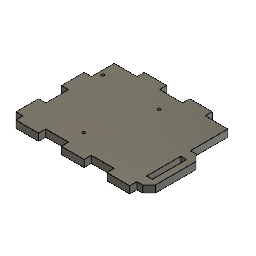
Right Side (Autodesk Fusion 360 design; units mm, degrees)
Autodesk Fusion 360 part; units mm, degrees
sketch "Sketch1" plane through (0, 0, 0) normal (0, 1, 0) x (1, 0, 0)
  line L0 (100, 38.5) -> (105, 38.5)
  line L1 (105, 38.5) -> (105, 8.5)
  line L2 (105, 8.5) -> (100, 8.5)
  line L3 (100, 8.5) -> (100, 38.5)
  line L4 (100, 0) -> (105, 0)
  line L5 (105, 0) -> (110.6569, 5.6569)
  line L6 (100, 47) -> (105, 47)
  line L7 (105, 47) -> (110.6569, 41.3431)
  line L8 (110.6569, 41.3431) -> (110.6569, 5.6569)
  line L9 (20, 0) -> (20, -6.35)
  line L10 (20, -6.35) -> (0, -6.35)
  line L11 (0, -6.35) -> (0, 0)
  line L12 (60, 0) -> (60, -6.35)
  line L13 (60, -6.35) -> (40, -6.35)
  line L14 (40, -6.35) -> (40, 0)
  line L15 (100, 0) -> (100, -6.35)
  line L16 (100, -6.35) -> (80, -6.35)
  line L17 (80, -6.35) -> (80, 0)
  line L18 (0, 0) -> (-6.35, 0)
  line L19 (-6.35, 0) -> (-6.35, 20)
  line L20 (-6.35, 20) -> (0, 20)
  line L21 (0, 40) -> (-6.35, 40)
  line L22 (-6.35, 40) -> (-6.35, 60)
  line L23 (-6.35, 60) -> (0, 60)
  line L24 (40, 80) -> (40, 86.35)
  line L25 (40, 86.35) -> (20, 86.35)
  line L26 (20, 86.35) -> (20, 80)
  line L27 (80, 80) -> (80, 86.35)
  line L28 (80, 86.35) -> (60, 86.35)
  line L29 (60, 86.35) -> (60, 80)
  line L30 (0, 20) -> (-6.35, 20)
  line L31 (-6.35, 20) -> (-6.35, 0)
  line L32 (-6.35, 0) -> (0, 0)
  line L33 (0, 0) -> (0, -6.35)
  line L34 (0, -6.35) -> (20, -6.35)
  line L35 (20, -6.35) -> (20, 0)
  line L36 (20, 0) -> (40, 0)
  line L37 (40, 0) -> (40, -6.35)
  line L38 (40, -6.35) -> (60, -6.35)
  line L39 (60, -6.35) -> (60, 0)
  line L40 (60, 0) -> (80, 0)
  line L41 (80, 0) -> (80, -6.35)
  line L42 (80, -6.35) -> (100, -6.35)
  line L43 (100, -6.35) -> (100, 0)
  line L44 (100, 0) -> (105, 0)
  line L45 (105, 0) -> (110.6569, 5.6569)
  line L46 (110.6569, 5.6569) -> (110.6569, 41.3431)
  line L47 (110.6569, 41.3431) -> (105, 47)
  line L48 (105, 47) -> (100, 47)
  line L49 (100, 47) -> (100, 80)
  line L50 (100, 80) -> (80, 80)
  line L51 (80, 80) -> (80, 86.35)
  line L52 (80, 86.35) -> (60, 86.35)
  line L53 (60, 86.35) -> (60, 80)
  line L54 (60, 80) -> (40, 80)
  line L55 (40, 80) -> (40, 86.35)
  line L56 (40, 86.35) -> (20, 86.35)
  line L57 (20, 86.35) -> (20, 80)
  line L58 (20, 80) -> (0, 80)
  line L59 (0, 80) -> (0, 60)
  line L60 (0, 60) -> (-6.35, 60)
  line L61 (-6.35, 60) -> (-6.35, 40)
  line L62 (-6.35, 40) -> (0, 40)
  line L63 (0, 40) -> (0, 20)
  line L64 (0, 20) -> (-6.35, 20)
  line L65 (-6.35, 20) -> (-6.35, 0)
  line L66 (-6.35, 0) -> (0, 0)
  circle A0 centre (4, 66) radius 1.25
  circle A1 centre (54.7, 64.7) radius 1.25
  circle A2 centre (39.5, 13.9) radius 1.25
  dimension "d1" = 80
  dimension "d2" = 100
  dimension "d3" = 5
  dimension "d4" = 30
  dimension "d7" = 5
  dimension "d8" = 8
  dimension "d10" = 45
  dimension "d11" = 5
  dimension "d12" = 8.5
  dimension "d13" = 8
  dimension "d14" = 45
  dimension "d17" = 20
  dimension "d18" = 6.35
  dimension "d19" = 6.35
  dimension "d20" = 20
  dimension "d21" = 40
  dimension "d22" = 6.35
  dimension "d23" = 20
  dimension "d24" = 20
  dimension "d25" = 6.35
  dimension "d26" = 20
  dimension "d27" = 6.35
  dimension "d28" = 20
  dimension "d29" = 20
  dimension "d32" = 6.35
  dimension "d33" = 20
  dimension "d34" = 6.35
  dimension "d35" = 20
  dimension "d36" = 20
  dimension "d40" = 6.35
  dimension "d41" = 6.35
  dimension "d42" = 8.5
  dimension "d43" = 5.6569
  dimension "d47" = 6.35
  dimension "d48" = 6.35
  dimension "d49" = 6.35
  dimension "d51" = 80
  dimension "d53" = 90
  dimension "d54" = 40
  dimension "d55" = 20
  dimension "d56" = 20
  dimension "d57" = 2.5
  dimension "d58" = 2.5
  dimension "d59" = 2.5
  dimension "d61" = 15.2
  dimension "d62" = 1.3
  dimension "d63" = 50.8
  dimension "d64" = 50.7
  measures "d1" distance of L11.end
  measures "d2" distance of L11.end
  measures "d4" distance of L11.end
  measures "d7" distance of L11.end
  measures "d8" distance of L11.end
  measures "d10" angle of L1 L5
  measures "d12" distance of L0 L6
  measures "d14" angle of L1 L7
  measures "d18" distance of L11.end
  measures "d19" distance of L11.end
  measures "d21" distance of L11 L14
  measures "d24" distance of L12 L17
  measures "d25" distance of L11.end
  measures "d27" distance of L9.start
  measures "d28" distance of L21 L23
  measures "d29" distance of L20 L21
  measures "d36" distance of L24 L29
  measures "d40" distance of L34 L36
  measures "d41" distance of L13 L40
  measures "d42" distance of L2 L44
  measures "d43" distance of L1 L8
  measures "d47" distance of L42 L44
  measures "d48" distance of L19 L63
  measures "d49" distance of L59 L61
  measures "d51" distance of L40 L50
  measures "d53" angle of L49 L50
  measures "d54" distance of L55 L59
  measures "d55" distance of L11.end
  measures "d56" distance of L23 L54
  measures "d57" diameter of A0
  measures "d58" diameter of A1
  measures "d59" diameter of A2
  measures "d61" distance of L11.end
  measures "d62" distance of L11.end
  measures "d63" distance of L11.end
  measures "d64" distance of L11.end
extrude "Extrude5" add sketch "Sketch1" along normal blind 6.35
extrude "Extrude4" [suppressed]
extrude "Extrude3" [suppressed]
extrude "Extrude2" [suppressed]
extrude "Extrude1" [suppressed]
equation "d12 = ( 17 / 2 ) * 1 mm"
